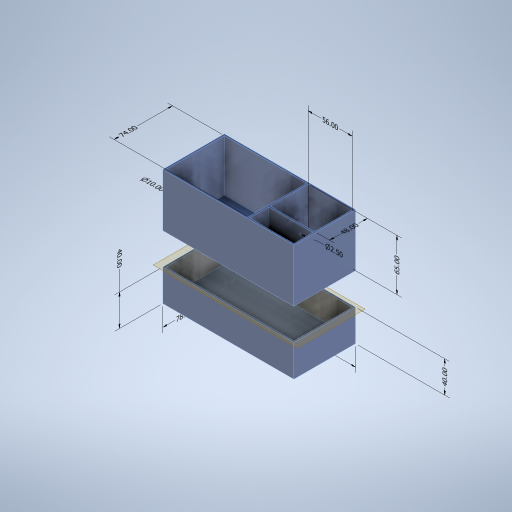
# Autodesk Inventor part: Capsula
Saved by Autodesk Inventor 2023 (Build 270158000, 158)
## iProperties
Created: 2023-03-19
Part Number: Capsula
Material: Plástico PET
Document SubType Name: Modeling
Designer: sergi
Density: 1.541 g/cm^3
Appearance: Satinado con motas - Azul
Author: sergi
Autodesk Inventor part; units mm, degrees
ref_plane "YZ Plane" through (0, 0, 0) normal (1, 0, 0) x (0, 1, 0)
ref_plane "XY Plane" through (0, 0, 0) normal (0, 0, 1) x (1, 0, 0)
sketch "Boceto1" plane through (0, 0, 0) normal (0, 1, 0) x (-1, 0, 0)
  line L0 (-41.5, 19.5) -> (41.5, 19.5)
  line L1 (41.5, 19.5) -> (41.5, -19.5)
  line L2 (41.5, -19.5) -> (-41.5, -19.5)
  line L3 (-41.5, -19.5) -> (-41.5, 19.5)
  line L4 (-41.5, 19.5) -> (41.5, -19.5) construction
  line L5 (41.5, 19.5) -> (-41.5, -19.5) construction
  line L6 (-40.5, 18.5) -> (40.5, 18.5)
  line L7 (40.5, 18.5) -> (40.5, -18.5)
  line L8 (40.5, -18.5) -> (-40.5, -18.5)
  line L9 (-40.5, -18.5) -> (-40.5, 18.5)
  line L10 (-40.5, 18.5) -> (40.5, -18.5) construction
  line L11 (40.5, 18.5) -> (-40.5, -18.5) construction
  point P0 (0, 0)
  dimension "d0" = 83
  dimension "d1" = 39
  dimension "d2" = 1
  dimension "d3" = 1
  constraints: 24 end point, 4 midpoint, 4 parallel, 2 horizontal, 2 perpendicular
  measures "d0" distance of L1.end L2.end
  measures "d1" distance of L0.end L1.end
  measures "d2" distance between parallel lines of L1 L7
  measures "d3" distance between parallel lines of L2 L8
extrude "Extrusión1" add sketch "Boceto1" along normal blind 3 contours L6 L7 L8 L9
extrude "Extrusión2" add sketch "Boceto1" along normal blind 20
sketch "Boceto2" plane through (0, 20, 0) normal (0, 1, 0) x (1, 0, 0)
  line L0 (41.5, 19.5) -> (-41.5, 19.5) projected
  line L1 (41.5, -19.5) -> (-41.5, -19.5)
  line L2 (-41.5, -19.5) -> (-41.5, 19.5)
  line L3 (-41.5, 19.5) -> (41.5, 19.5)
  line L4 (41.5, 19.5) -> (41.5, -19.5)
  line L5 (41.5, -19.5) -> (-41.5, 19.5) construction
  line L6 (-41.5, -19.5) -> (41.5, 19.5) construction
  line L7 (35.5, -13.5) -> (-35.5, 13.5) construction
  line L8 (-35.5, -13.5) -> (35.5, 13.5) construction
  point P0 (0, 0)
  constraints: 16 end point, 4 midpoint, 2 parallel, 1 horizontal, 1 perpendicular
extrude "Extrusión3" add sketch "Boceto2" along normal blind 1
sketch "Boceto3" plane through (0, 21, 0) normal (0, 1, 0) x (1, 0, 0)
  point P0 (0, 0)
sketch "Boceto4" plane through (0, 21, 0) normal (0, 1, 0) x (1, 0, 0)
  line L0 (-41.5, 19.5) -> (-41.5, -19.5) projected
  line L1 (41.5, -19.5) -> (-41.5, -19.5)
  line L2 (-41.5, -19.5) -> (-41.5, 19.5)
  line L3 (-41.5, 19.5) -> (41.5, 19.5)
  line L4 (41.5, 19.5) -> (41.5, -19.5)
  line L5 (41.5, -19.5) -> (-41.5, 19.5) construction
  line L6 (-41.5, -19.5) -> (41.5, 19.5) construction
  line L7 (40.5, -18.5) -> (-40.5, -18.5)
  line L8 (-40.5, -18.5) -> (-40.5, 18.5)
  line L9 (-40.5, 18.5) -> (40.5, 18.5)
  line L10 (40.5, 18.5) -> (40.5, -18.5)
  line L11 (40.5, -18.5) -> (-40.5, 18.5) construction
  line L12 (-40.5, -18.5) -> (40.5, 18.5) construction
  point P0 (0, 0)
  point P1 (-41.5, -19.5)
  dimension "d21" = 1
  dimension "d22" = 1
  constraints: 24 end point, 4 midpoint, 4 parallel, 2 horizontal, 2 perpendicular
  measures "d21" distance between parallel lines of L0 L8
  measures "d22" distance between parallel lines of L3 L9
extrude "Extrusión4" add sketch "Boceto4" along normal blind 32.5
ref_plane "Work Plane1" through (0, 20, 0) normal (0, 1, 0) x (-1, 0, 0)
split body "Split1" result two bodies by plane through (0, 20, 0) normal (0, 1, 0) first body at (13.5, 20.5, 6.1667)
move or copy body "Move1" bodies to move or copy 2 copy no translate (0, 20, 0)
sketch "Boceto6" plane through (-40.5, 41, -18.5) normal (0, 1, 0) x (1, 0, 0)
  line L0 (81, 0) -> (81, -37) projected
  line L1 (81, 0) -> (0, 0) projected
  line L2 (81, -37) -> (53, -37)
  line L3 (53, -37) -> (53, 0)
  line L4 (53, 0) -> (81, 0)
  line L5 (81, 0) -> (81, -37)
  line L6 (0, -37) -> (81, -37) projected
  line L7 (81, -37) -> (52, -37)
  line L8 (52, -37) -> (52, 0)
  line L9 (52, 0) -> (81, 0)
  line L10 (81, 0) -> (81, -37)
  point P0 (40.5, -18.5)
  dimension "d42" = 28
  dimension "d43" = 29
  constraints: 16 end point, 4 parallel, 2 horizontal, 2 perpendicular, 2 point on line
  measures "d42" distance of L3.end L4.end
  measures "d43" distance of L8.end L9.end
extrude "Extrusión6" add sketch "Boceto6" along normal blind 32.5 contours L3 L6 L8 L1 bodies 2
sketch "Boceto7" plane through (40.5, 41, 18.5) normal (0, 1, 0) x (1, 0, 0)
  line L0 (-28, 37) -> (0, 37) projected
  line L1 (-28, 37) -> (-28, 0) projected
  line L2 (0, 37) -> (-28, 37)
  line L3 (-28, 37) -> (-28, 12)
  line L4 (-28, 12) -> (0, 12)
  line L5 (0, 12) -> (0, 37)
  line L6 (0, 37) -> (-28, 37)
  line L7 (-28, 37) -> (-28, 13)
  line L8 (-28, 13) -> (0, 13)
  line L9 (0, 13) -> (0, 37)
  point P0 (-40.5, 18.5)
  point P1 (0, 13)
  point P2 (-28, 13)
  dimension "d49" = 25
  dimension "d50" = 1
  constraints: 16 end point, 4 parallel, 2 horizontal, 2 perpendicular, 2 point on line
  measures "d49" distance of L4.end L0.end
  measures "d50" distance between parallel lines of L4 L8
extrude "Extrusión7" add sketch "Boceto7" along normal blind 32.5 contours L8 L5 L4 L1 bodies 2
sketch "Boceto8" plane through (12.5, 41, -18.5) normal (0, 1, 0) x (1, 0, 0)
  circle A0 centre (14, -12.5) radius 7
  line L0 (28, 0) -> (28, -24) projected
  line L1 (28, -24) -> (0, -24) projected
  circle A1 centre (14, -12.5) radius 8
  point P0 (-12.5, -18.5)
  dimension "d53" = 14
  dimension "d54" = 14
  dimension "d55" = 24
  dimension "d56" = 11.5
  dimension "d57" = 16
  constraints: 2 centre point, 1 coincident
  measures "d53" diameter of A0
  measures "d54" distance from line of A0.centre L0
  measures "d55" distance of L0.start L0.end
  measures "d56" distance from line of L1 A0.centre
  measures "d57" diameter of A1
extrude "Extrusión8" add sketch "Boceto8" along normal blind 10 bodies 2
sketch "Boceto9" plane through (26.5, 41, -6) normal (0, 1, 0) x (1, 0, 0)
  circle A0 centre (0, -6) radius 0.575
  circle A1 centre (0, 0) radius 7 projected
  circle A2 centre (0, 6) radius 0.575
  point P0 (-26.5, -6)
  dimension "d60" = 1.15
  dimension "d61" = 6
  dimension "d62" = 1.15
  dimension "d63" = 6
  constraints: 2 centre point
  measures "d60" diameter of A0
  measures "d61" distance of A1.centre A0.centre
  measures "d62" diameter of A2
  measures "d63" distance of A1.centre A2.centre
extrude "Extrusión9" cut sketch "Boceto9" against normal blind 1 contours A0 | A2 bodies 2
sketch "Boceto10" plane through (12.5, 41, 6.5) normal (0, 0, 1) x (1, 0, 0)
  line L0 (0, 32.5) -> (0, 0) projected
  line L1 (0, 32.5) -> (20, 32.5)
  line L2 (0, 32.5) -> (28, 32.5) projected
  line L3 (20, 32.5) -> (20, 27.5)
  circle A0 centre (20, 27.5) radius 0.625
  line L4 (28, 0) -> (28, 32.5) projected
  point P0 (-12.5, -41)
  dimension "d69" = 20
  dimension "d70" = 5
  dimension "d71" = 1.25
  dimension "d81" = 8
  constraints: 4 end point, 1 centre point, 1 coincident, 1 point on line, 1 vertical
  measures "d69" distance of L0.start L1.end
  measures "d70" distance of L1.end L3.end
  measures "d71" diameter of A0
  measures "d81" distance from line of L4 L3.end
extrude "Extrusión10" cut sketch "Boceto10" against normal blind 1 bodies 2
scale "Escala1" factors (2, 2, 2) then translate (0, -40, 0) bodies 2 3
sketch "Boceto11" plane through (-81, 42, 37) normal (0, 1, 0) x (1, 0, 0)
  line L0 (0, 74) -> (0, 0) projected
  line L1 (0, 37) -> (30, 37)
  circle A0 centre (30, 37) radius 5
  point P0 (81, 37)
  dimension "d77" = 30
  dimension "d78" = 10
  constraints: 2 end point, 1 centre point, 1 coincident, 1 horizontal, 1 midpoint
  measures "d77" distance of L1.start L1.end
  measures "d78" diameter of A0
extrude "Extrusión11" cut sketch "Boceto11" against normal blind 10 bodies 2
body "Solid2"
body "Solid3"
